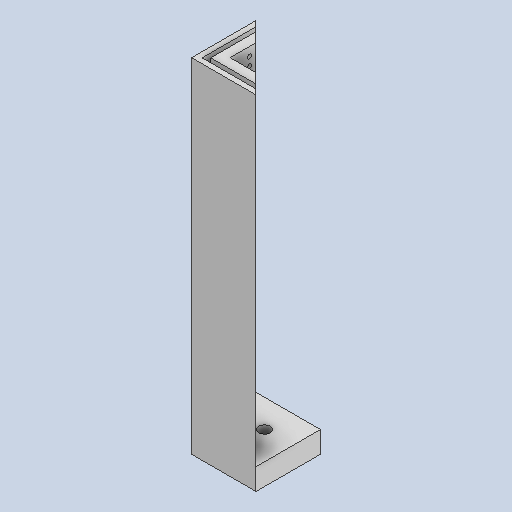
# Autodesk Inventor part: nohy
Saved by Autodesk Inventor 2025 (Build 290162000, 162)
## iProperties
Created: 2025-04-22
Part Number: nohy
Material: Generic
Document SubType Name: Sheet Metal
Designer: Pravoslav
Density: 1 g/cm^3
Sheet Metal Rule: Default_mm
Appearance: Default
Author: Pravoslav
Autodesk Inventor part; units mm, degrees
ref_plane "YZ Plane" through (0, 0, 0) normal (1, 0, 0) x (0, 1, 0)
ref_plane "XZ Plane" through (0, 0, 0) normal (0, 1, 0) x (-1, 0, 0)
ref_plane "XY Plane" through (0, 0, 0) normal (0, 0, 1) x (1, 0, 0)
sketch "Sketch1" plane through (0, 0, 0) normal (0, 1, 0) x (-1, 0, 0)
  line L0 (0, 0) -> (30, 0)
  line L1 (30, 0) -> (30, 30)
  line L2 (30, 30) -> (0, 30)
  line L3 (0, 30) -> (0, 0)
  circle A0 centre (13, 13) radius 2.65
  dimension "d0" = 30
  dimension "d1" = 30
  dimension "d2" = 5.3
  dimension "d3" = 17
  dimension "d4" = 17
  constraints: 8 end point, 2 parallel, 1 centre point, 1 horizontal, 1 perpendicular
  measures "d0" distance of L2.end L1.end
  measures "d1" distance of L1.end L0.end
  measures "d2" diameter of A0
  measures "d3" distance from line of L2 A0.centre
  measures "d4" distance from line of L1 A0.centre
extrude "Extrusion1" add sketch "Sketch1" along normal blind 10
sketch "Sketch2" plane through (0, 10, 0) normal (0, 1, 0) x (1, 0, 0)
  line L0 (-30, 0) -> (-30, -30) projected
  line L1 (-30, -30) -> (0, -30) projected
  line L2 (-30, 0) -> (0, -30)
  line L3 (0, -30) -> (-30, -30)
  line L4 (-30, -30) -> (-30, 0)
  line L5 (-27.4867, -2.5133) -> (-27.4867, -27.6058)
  line L6 (-27.4867, -27.6058) -> (-2.3942, -27.6058)
  line L7 (-4.3942, -25.6058) -> (-25.4867, -25.6058)
  line L8 (-25.4867, -25.6058) -> (-25.4867, -4.5133)
  line L9 (-21.0431, -8.9569) -> (-21.0431, -21.0431)
  line L10 (-21.0431, -21.0431) -> (-8.9569, -21.0431)
  point P0 (0, 0)
  dimension "d7" = 2
  dimension "d9" = 2
  constraints: 18 end point, 6 point on line, 4 perpendicular, 2 vertical, 1 collinear, 1 horizontal
  measures "d7" distance between parallel lines of L7 L6
  measures "d9" distance between parallel lines of L5 L8
extrude "Extrusion2" add sketch "Sketch2" along normal blind 150 contours L2 L5 L6 L1 L0 | L2 L9 L10 L7 L8
sketch "Sketch3" plane through (-21.0431, 10, 21.0431) normal (1, 0, 0) x (0, 0, -1)
  circle A0 centre (9.0861, 4) radius 1
  circle A1 centre (9.0861, 8) radius 1
  circle A2 centre (9.0861, 12) radius 1
  line L0 (-8.9569, 0) -> (21.0431, 0) projected
  line L1 (12.0861, 0) -> (12.0861, 150) projected
  circle A3 centre (9.0861, 67.9347) radius 1
  circle A4 centre (9.0861, 71.9347) radius 1
  circle A5 centre (9.0861, 75.9347) radius 1
  circle A6 centre (9.0861, 138) radius 1
  circle A7 centre (9.0861, 142) radius 1
  circle A8 centre (9.0861, 146) radius 1
  line L2 (0, 150) -> (12.0861, 150) projected
  point P0 (21.0431, -10)
  dimension "d12" = 2
  dimension "d13" = 2
  dimension "d14" = 2
  dimension "d15" = 4
  dimension "d16" = 4
  dimension "d18" = 12
  dimension "d19" = 3
  dimension "d20" = 3
  dimension "d21" = 3
  dimension "d22" = 2
  dimension "d23" = 2
  dimension "d24" = 2
  dimension "d25" = 4
  dimension "d26" = 4
  dimension "d27" = 3
  dimension "d28" = 2
  dimension "d29" = 2
  dimension "d30" = 2
  dimension "d31" = 4
  dimension "d32" = 4
  dimension "d33" = 4
  dimension "d34" = 3
  constraints: 9 centre point
  measures "d12" diameter of A0
  measures "d13" diameter of A1
  measures "d14" diameter of A2
  measures "d15" distance of A1.centre A0.centre
  measures "d16" distance of A2.centre A1.centre
  measures "d18" distance from line of L0 A2.centre
  measures "d19" distance from line of L1 A2.centre
  measures "d20" distance from line of L1 A1.centre
  measures "d21" distance from line of L1 A0.centre
  measures "d22" diameter of A3
  measures "d23" diameter of A4
  measures "d24" diameter of A5
  measures "d25" distance of A4.centre A3.centre
  measures "d26" distance of A5.centre A4.centre
  measures "d27" distance from line of L1 A5.centre
  measures "d28" diameter of A6
  measures "d29" diameter of A7
  measures "d30" diameter of A8
  measures "d31" distance of A7.centre A6.centre
  measures "d32" distance of A8.centre A7.centre
  measures "d33" distance from line of L2 A8.centre
  measures "d34" distance from line of L1 A8.centre
extrude "Extrusion3" cut sketch "Sketch3" against normal blind 150
equation "\"BendRadius\" = Thickness"
equation "\"BendReliefWidth\" = Thickness"
equation "\"BendReliefDepth\" = 0.5 * Thickness"
equation "\"CornerReliefSize\" = 4 * Thickness"
equation "\"MinimumRemnant\" = 2 * Thickness"
equation "\"TransitionRadius\" = BendRadius"
equation "\"JacobiRadiusSize\" = BendRadius"
equation "\"GapSize\" = Thickness"
equation "\"Thickness\" = 0.5"
body "Solid1"
